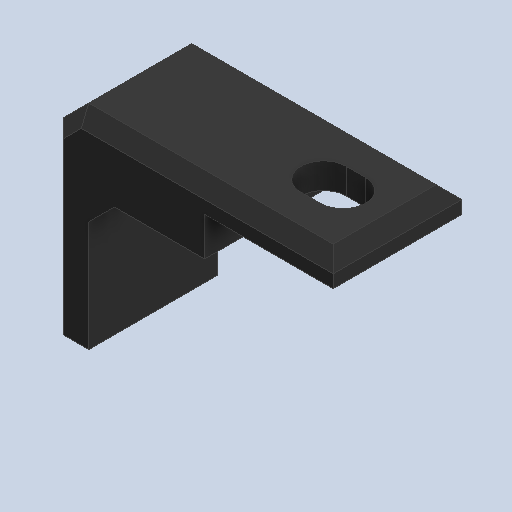
# Autodesk Inventor part: Connector_Stop
Saved by Autodesk Inventor 2022 (Build 260153000, 153)
## iProperties
Created: 2021-01-21
Part Number: Connector_Stop
Material: Generic
Document SubType Name: Modeling
Designer: Viktor
Density: 1 g/cm^3
Appearance: Default
Author: Viktor
## iProperties of the stored document _3DPrint.ipt
Created: 2021-01-26
Part Number: _3DPrint
Material: Generic
Document SubType Name: Modeling
Designer: Viktor
Density: 1 g/cm^3
Appearance: Default
Author: Viktor
Autodesk Inventor part; units mm, degrees
ref_plane "YZ Plane" through (0, 0, 0) normal (1, 0, 0) x (0, 1, 0)
ref_plane "XZ Plane" through (0, 0, 0) normal (0, 1, 0) x (-1, 0, 0)
ref_plane "XY Plane" through (0, 0, 0) normal (0, 0, 1) x (1, 0, 0)
sketch "Sketch1" plane through (0, 0, 0) normal (0, 0, 1) x (1, 0, 0)
  line L0 (0, 0) -> (-22, 0)
  line L1 (-22, 0) -> (-22, -15.6)
  line L2 (-22, -15.6) -> (-19, -15.6)
  line L3 (-19, -15.6) -> (-19, -5)
  line L4 (-19, -5) -> (-10, -5)
  line L5 (-10, -5) -> (-10, -2)
  line L6 (-10, -2) -> (0, -2)
  line L7 (0, -2) -> (0, 0)
  dimension "d0" = 2
  dimension "d1" = 10
  dimension "d2" = 3
  dimension "d3" = 9
  dimension "d4" = 3
  dimension "d5" = 10.6
  constraints: 16 end point, 7 perpendicular, 1 horizontal
  measures "d0" distance between parallel lines of L0 L6
  measures "d1" distance between parallel lines of L5 L7
  measures "d2" distance of L4.end L5.end
  measures "d3" distance of L3.end L4.end
  measures "d4" distance between parallel lines of L3 L1
  measures "d5" distance between parallel lines of L4 L2
extrude "Extrusion1" add sketch "Sketch1" along normal blind 10
chamfer "Chamfer1" distance 2 angle 45 1 edges at (-19, -5, 5)
sketch "Sketch2" plane through (-22, 0, 0) normal (0, 1, 0) x (1, 0, 0)
  line L0 (12, 0) -> (12, -10) projected
  line L1 (16.25, -5) -> (17.75, -5) construction
  line L2 (16.25, -6.75) -> (17.75, -6.75)
  line L3 (17.75, -3.25) -> (16.25, -3.25)
  arc A0 (16.25, -3.25) -> (16.25, -6.75) centre (16.25, -5) ccw
  arc A1 (17.75, -6.75) -> (17.75, -3.25) centre (17.75, -5) ccw
  point P0 (22, 0)
  point P1 (17, -5)
  dimension "d11" = 1.75
  dimension "d12" = 1.5
  dimension "d13" = 5
  constraints: 8 end point, 4 point on circle, 4 tangent, 2 centre point, 1 horizontal, 1 midpoint, 1 parallel
  measures "d11" radius of A1
  measures "d12" distance of L3.start L3.end
  measures "d13" distance from line of L0 point (17, -5)
extrude "Extrusion2" cut sketch "Sketch2" against normal through all
chamfer "Chamfer2" distance 2 angle 45 1 edges at (-22, 0, 5)
chamfer "Chamfer3" distance 1 angle 45 8 edges at (-10, 0, 10) (-10, 0, 0) (0, 0, 5) (-21, -1, 10) (-22, -8.8, 10) (-21, -1, 0) (-22, -8.8, 0) (-22, -15.6, 5)
body "Solid1"
